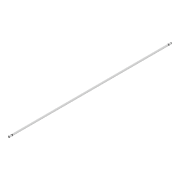
# Autodesk Inventor part: union
Saved by Autodesk Inventor 2021 (Build 250183000, 183)
## iProperties
Created: 2021-04-19
Part Number: union
Material: Genérico
Document SubType Name: Modeling
Designer: carlo
Density: 1 g/cm^3
Appearance: Valor por defecto
Author: carlo
Autodesk Inventor part; units mm, degrees
ref_plane "YZ Plane" through (0, 0, 0) normal (1, 0, 0) x (0, 1, 0)
ref_plane "XZ Plane" through (0, 0, 0) normal (0, 1, 0) x (-1, 0, 0)
ref_plane "XY Plane" through (0, 0, 0) normal (0, 0, 1) x (1, 0, 0)
sketch "Boceto1" plane through (0, 0, 0) normal (0, 0, 1) x (1, 0, 0)
  circle A0 centre (0, 0) radius 2.5
  dimension "d1" = 5
  constraints: 1 centre point, 1 coincident
  measures "d1" diameter of A0
extrude "Extrusión1" add sketch "Boceto1" along normal blind 513
sketch "Boceto2" plane through (0, 0, 0) normal (1, 0, 0) x (0, 1, 0)
  line L0 (0, 0) -> (0, 8.92)
  line L1 (0, 8.92) -> (-2.5, 8.92)
  line L2 (-2.5, 0) -> (-2.5, 513) projected
  line L3 (-2.5, 0) -> (-2.5, 513) projected
  line L4 (-2.5, 8.42) -> (-2, 8.42)
  line L5 (-2, 8.42) -> (-2, 9.42)
  line L6 (-2, 9.42) -> (-2.5, 9.42)
  line L7 (-2.5, 9.42) -> (-2.5, 8.42)
  dimension "d4" = 8.92
  constraints: 12 end point, 2 horizontal, 2 parallel, 2 point on line, 1 coincident, 1 perpendicular, 1 vertical
  measures "d4" distance of L0.start L0.end
revolve "Revolución1" cut sketch "Boceto2" angle 360 about axis through (0, 0, 0) along (0, 0, 1)
sketch "Boceto3" plane through (0, 0, 0) normal (1, 0, 0) x (0, 1, 0)
  line L0 (2.5, 513) -> (-2.5, 513) projected
  line L1 (0, 513) -> (0, 503.5)
  line L2 (0, 503.5) -> (-2.5, 503.5)
  line L3 (-2.5, 9.42) -> (-2.5, 513) projected
  line L4 (-2.5, 503.5) -> (-2, 503.5)
  line L5 (-2, 503.5) -> (-2, 503)
  line L6 (-2, 503) -> (-2.5, 503)
  line L7 (-2.5, 503) -> (-2.5, 503.5)
  line L8 (-2.5, 503.5) -> (-2, 503.5)
  line L9 (-2, 503.5) -> (-2, 504)
  line L10 (-2, 504) -> (-2.5, 504)
  line L11 (-2.5, 504) -> (-2.5, 503.5)
  point P0 (0, 0)
  dimension "d8" = 9.5
  dimension "d9" = 0.5
  dimension "d10" = 0.5
  dimension "d11" = 0.5
  dimension "d12" = 0.5
  constraints: 20 end point, 4 parallel, 3 horizontal, 2 perpendicular, 1 midpoint, 1 point on line, 1 vertical
  measures "d8" distance of L1.start L1.end
  measures "d9" distance of L5.end L6.end
  measures "d10" distance of L4.end L5.end
  measures "d11" distance of L10.end L9.end
  measures "d12" distance of L9.end L8.end
revolve "Revolución2" cut sketch "Boceto3" angle 360 about axis through (0, 0, 513) along (0, 0, -1) contours L10 L9 L2 L3 | L5 L6 L3 L2
